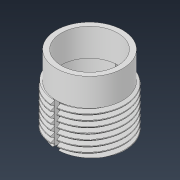
# Autodesk Inventor part: bottomPiece
Saved by Autodesk Inventor 2022 (Build 260153000, 153)
## iProperties
Created: 2022-07-02
Part Number: bottomPiece
Material: Generic
Document SubType Name: Modeling
Designer: User
Density: 1 g/cm^3
Appearance: Default
Author: User
## iProperties of the stored document bottomPiece_3DPrint.ipt
Created: 2022-07-04
Part Number: bottomPiece_3DPrint
Material: Generic
Document SubType Name: Modeling
Designer: User
Density: 1 g/cm^3
Appearance: Default
Author: User
Autodesk Inventor part; units mm, degrees
ref_plane "YZ Plane" through (0, 0, 0) normal (1, 0, 0) x (0, 1, 0)
ref_plane "XZ Plane" through (0, 0, 0) normal (0, 1, 0) x (-1, 0, 0)
ref_plane "XY Plane" through (0, 0, 0) normal (0, 0, 1) x (1, 0, 0)
sketch "Sketch1" plane through (0, 0, 0) normal (0, 1, 0) x (-1, 0, 0)
  circle A0 centre (0, 0) radius 9.9
  circle A1 centre (0, 0) radius 13
  dimension "d0" = 19.8
  dimension "d1" = 26
  constraints: 2 centre point, 2 coincident
  measures "d0" diameter of A0
  measures "d1" diameter of A1
extrude "Extrusion1" add sketch "Sketch1" along normal blind 15
chamfer "Chamfer1" distance 1 angle 45 1 edges at (13, 0, 0)
sketch "Sketch12" plane through (0, 0, 0) normal (0, -1, 0) x (1, 0, 0)
  circle A0 centre (0, 0) radius 9.9 projected
  circle A1 centre (0, 0) radius 12 projected
  circle A2 centre (0, 0) radius 10.2
  dimension "d74" = 20.4
  constraints: 1 centre point, 1 coincident
  measures "d74" diameter of A2
extrude "Extrusion3" add sketch "Sketch12" along normal blind 10 contours A1
sketch "Sketch11" plane through (0, 15, 0) normal (1, 0, 0) x (0, 0, 1)
  line L0 (13, 0) -> (13, 15)
  line L1 (13, 15) -> (11.5171, 15)
  line L2 (11.5171, 15) -> (11.5171, 0)
  line L3 (11.5171, 0) -> (13, 0)
  line L4 (0, -3) -> (0, 18) projected
  constraints: 8 end point
revolve "Revolution6" add sketch "Sketch11" angle 360 about axis through (0, 15, 0) along (0, -1, 0) separate body
thread "M28x2" size "M28x2" class "6g" standard "ANSI Metric M Profile" full length
sketch "Sketch10" plane through (0, 15, 0) normal (1, 0, 0) x (0, 0, 1)
  line L0 (13, 0) -> (13, 15)
  line L1 (13, 15) -> (11.5171, 15)
  line L2 (11.5171, 15) -> (11.5171, 0)
  line L3 (11.5171, 0) -> (13, 0)
  line L4 (0, -3) -> (0, 18) projected
  constraints: 8 end point
revolve "Revolution5" cut sketch "Sketch10" angle 360 about axis through (0, 15, 0) along (0, -1, 0) bodies 1
sketch "Sketch9" plane through (0, 15, 0) normal (-1, 0, 0) x (0, -1, 0)
  line L0 (-1.1668, -11.6184) -> (-1.0001, -11.6184) construction
  line L1 (0.1666, -12.899) -> (-0.0001, -13.2192) construction
  line L2 (-2.0001, -13.2192) -> (-2.1668, -12.899) construction
  line L3 (-0.8334, -11.6184) -> (-1.0001, -11.2982) construction
  line L4 (-1.0001, -11.2982) -> (-1.1668, -11.6184) construction
  line L5 (-2.0001, -13.2192) -> (-1.8334, -12.899) construction
  line L6 (-0.8334, -11.6184) -> (-0.1668, -12.899)
  line L7 (-2.1668, -12.899) -> (-1.8334, -12.899) construction
  arc A0 (-2.1668, -12.899) -> (-2.0001, -13.0002) centre (-2.0001, -12.8123) ccw construction
  line L8 (0.1666, -12.899) -> (-0.1668, -12.899) construction
  line L9 (-2.0001, -13.2192) -> (-2.0001, -12.899) construction
  line L10 (-0.0001, -13.2192) -> (-0.0001, -12.899) construction
  line L11 (-1.0001, -11.2982) -> (-1.0001, -11.5172) construction
  line L12 (-2.0001, -13.0002) -> (-0.0001, -13.0002)
  arc A1 (-2.0001, -13.0002) -> (-1.8334, -12.899) centre (-2.0001, -12.8123) ccw
  line L13 (-0.1668, -12.899) -> (-0.0001, -13.2192) construction
  line L14 (-1.8334, -12.899) -> (-1.1668, -11.6184)
  line L15 (-0.0001, -0.0002) -> (-0.0001, 0.0177)
  line L16 (-0.0001, 0.0177) -> (-0.0001, -0.0002)
  line L17 (-0.0001, -0.0002) -> (0.0334, -0.0002)
  arc A2 (-0.1668, -12.899) -> (-0.0001, -13.0002) centre (-0.0001, -12.8123) ccw
  arc A3 (-0.0001, -13.0002) -> (0.1666, -12.899) centre (-0.0001, -12.8123) ccw construction
  arc A4 (-1.0001, -11.5172) -> (-1.1668, -11.6184) centre (-1.0001, -11.7051) ccw
  arc A5 (-0.8334, -11.6184) -> (-1.0001, -11.5172) centre (-1.0001, -11.7051) ccw
  line L18 (-1.0001, -11.5172) -> (-1.0001, -11.6184) construction
  line L19 (-1.0001, -11.6184) -> (-0.8334, -11.6184) construction
  dimension "d53" = 55
  dimension "d54" = 0.3202
  dimension "d55" = 0.3202
  dimension "Sketch9_ThreadOffset" = 0
  dimension "Sketch9_MajorRadius" = 13
  dimension "d58" = 2
  dimension "Sketch9_MinorRadius" = 11.5171
  constraints: 40 end point, 12 point on circle, 10 parallel, 8 tangent, 6 centre point, 6 collinear, 2 midpoint, 2 point on line, 1 horizontal, 1 perpendicular, 3 other
  measures "d53" angle of L6 L14
  measures "d54" distance of L3.end L0.end
  measures "d55" distance of L1.end L10.end
  measures "Sketch9_ThreadOffset" distance between parallel lines of L15 L10
  measures "Sketch9_MajorRadius" distance from line of L12 L15.start
  measures "d58" distance from line of L1.end L9
  measures "Sketch9_MinorRadius" distance edge to line of A5 L17
coil "Coil3" sketch "Sketch9" operation cut axis through (0, 15, 0) along (0, -1, 0) pitch 2.002 turns 9.490509 hand right bodies 2
sketch "Sketch8" plane through (0, 0, 0) normal (0, 1, 0) x (-1, 0, 0)
  circle A0 centre (0, 0) radius 13
  line L0 (0, 0) -> (12.9505, -1.133)
  line L1 (0, 0) -> (13, 0) construction
  line L2 (0, 0) -> (12.9505, 1.133)
  line L3 (0, -2.676) -> (0, 3.4077) construction
  line L4 (0, 0) -> (-12.9505, -1.133)
  line L5 (0, 0) -> (-12.9505, 1.133)
  dimension "d46" = 26
  dimension "d47" = 5
  constraints: 12 end point, 3 symmetric about line, 1 coincident, 1 equal length, 1 horizontal, 1 vertical, 3 other
  measures "d47" angle of L0 L1
extrude "slot" cut sketch "Sketch8" along normal through all contours A0 L0 L2 | L5 L4 A0 bodies 1 2
sketch "Sketch13" plane through (0, 0, 0) normal (1, 0, 0) x (0, 1, 0)
  line L0 (-10, 10.2) -> (0, 10.2) projected
  line L1 (15, 9.9) -> (0, 9.9) projected
  line L2 (0, 10.2) -> (15, 9.9)
  line L3 (0, 10.2) -> (0, 9.9)
  line L4 (0, 0) -> (1.7608, 0) construction
  constraints: 6 end point
revolve "Revolution7" cut sketch "Sketch13" angle 360 about axis through (0, 0, 0) along (0, 1, 0) bodies 1
equation "\"d53\" = d60"
equation "\"d54\" = 0.160083 * Sketch9_Pitch"
equation "\"d55\" = 0.160083 * Sketch9_Pitch"
equation "\"d58\" = Sketch9_Pitch"
equation "\"d13\" = 55deg"
equation "\"Sketch2_Pitch\" = 1.5"
equation "\"d34\" = 55deg"
equation "\"Sketch5_Pitch\" = 2"
equation "\"d60\" = 55deg"
equation "\"Sketch9_Pitch\" = 2"
body "Solid1"
body "Solid4"
